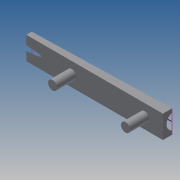
# Autodesk Inventor part: 滑軌3
Saved by Autodesk Inventor 2015 (Build 190159000, 159)
## iProperties
Created: 2018-01-06
Part Number: 滑軌3
Material: 一般
Document SubType Name: Modeling
Designer: user
Density: 1 g/cm^3
Appearance: 預設
Author: user
Autodesk Inventor part; units mm, degrees
ref_plane "YZ Plane" through (0, 0, 0) normal (1, 0, 0) x (0, 1, 0)
ref_plane "XZ Plane" through (0, 0, 0) normal (0, 1, 0) x (-1, 0, 0)
ref_plane "XY Plane" through (0, 0, 0) normal (0, 0, 1) x (1, 0, 0)
sketch "草圖1" plane through (0, 0, 0) normal (0, 0, 1) x (1, 0, 0)
  line L0 (0, 0) -> (150, 4)
  line L1 (150, 4) -> (150, -6)
  line L2 (150, -6) -> (0, -6)
  line L3 (0, -6) -> (0, 0)
  dimension "d0" = 10
  dimension "d1" = 6
  dimension "d2" = 150
  constraints: 8 end point, 2 perpendicular, 1 vertical
  measures "d0" distance of L0.end L1.end
  measures "d1" distance of L2.end L0.start
  measures "d2" horizontal distance of L0.start L0.end
extrude "擠出1" add sketch "草圖1" along normal blind 25
sketch "草圖2" plane through (0, -6, 0) normal (0, -1, 0) x (1, 0, 0)
  circle A0 centre (50, 12.5) radius 5
  circle A1 centre (130, 12.5) radius 5
  line L0 (0, 25) -> (150, 25) projected
  line L1 (150, 0) -> (150, 25) projected
  point P0 (0, 0)
  dimension "d5" = 12.5
  dimension "d6" = 10
  dimension "d7" = 10
  dimension "d8" = 80
  dimension "d9" = 20
  constraints: 2 centre point, 1 horizontal alignment
  measures "d5" distance from line of L0 A1.centre
  measures "d6" diameter of A1
  measures "d7" diameter of A0
  measures "d8" distance of A1.centre A0.centre
  measures "d9" distance from line of L1 A1.centre
extrude "擠出2" add sketch "草圖2" along normal blind 21
sketch "草圖3" plane through (0, -6, 0) normal (-1, 0, 0) x (0, 0, 1)
  line L0 (0, 0) -> (0, 6) construction
  line L1 (0, 0) -> (25, 0) construction
  line L2 (25, 6) -> (25, 0) construction
  line L3 (0, 6) -> (25, 6) construction
  line L4 (21, 6) -> (4, 6)
  line L5 (0, 6) -> (25, 6) projected
  arc A0 (4.2386, 6) -> (20.7614, 6) centre (12.5, 8) ccw
  dimension "d23" = 17
  dimension "d25" = 2
  constraints: 4 point on line, 2 end point, 2 point on circle, 1 centre point, 1 collinear
  measures "d23" diameter of A0
  measures "d25" vertical distance of L2.start A0.centre
sketch "草圖4" plane through (150, -6, 0) normal (1, 0, 0) x (0, 0, -1)
  line L0 (-21.5, 11) -> (-3.5, 11)
  arc A0 (-21.275, 11) -> (-3.725, 11) centre (-12.5, 13) ccw
  line L1 (0, 10) -> (0, 0) projected
  dimension "d19" = 18
  dimension "d21" = 2
  dimension "d22" = 12.5
  constraints: 2 end point, 2 point on circle, 2 point on line, 1 centre point
  measures "d19" diameter of A0
  measures "d21" distance from line of L0 A0.centre
  measures "d22" distance from line of L1 A0.centre
sketch "草圖5" plane through (0, 0, 25) normal (-0.0267, 0.9996, 0) x (0.9996, 0.0267, 0)
  line L0 (150.0533, 25) -> (150.0533, 0) projected
  line L1 (150.0533, 12.5) -> (0, 12.5)
  line L2 (0, 25) -> (0, 0) projected
  constraints: 2 end point, 2 midpoint
loft "斷面混成2" cut profiles "草圖4", "草圖3"
